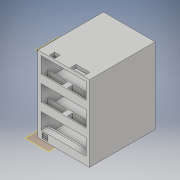
# Autodesk Inventor part: Relé - columnes tapa
Saved by Autodesk Inventor 2019 (Build 230136000, 136)
## iProperties
Created: 2018-08-23
Part Number: Relé - columnes tapa
Material: Genérico
Document SubType Name: Modeling
Designer: Albert Garangou Culebras
Density: 1 g/cm^3
Appearance: Valor por defecto
Author: Albert Garangou Culebras
Autodesk Inventor part; units mm, degrees
ref_plane "YZ Plane" through (0, 0, 0) normal (1, 0, 0) x (0, 1, 0)
ref_plane "XZ Plane" through (0, 0, 0) normal (0, 1, 0) x (-1, 0, 0)
ref_plane "XY Plane" through (0, 0, 0) normal (0, 0, 1) x (1, 0, 0)
ref_plane "Plano de trabajo1" through (0, 3, 0) normal (0, 1, 0) x (1, 0, 0)
ref_plane "Plano de trabajo2" through (4.2498, 73, -5.25) normal (0, 1, 0) x (1, 0, 0)
sketch "Boceto3" plane through (4.2498, 73, -5.25) normal (0, 1, 0) x (1, 0, 0)
  line L0 (37.7502, 51.75) -> (40.7502, 51.75)
  line L1 (-7.2498, -8.25) -> (40.7502, -8.25)
  line L2 (40.7502, -8.25) -> (40.7502, 51.75)
  line L3 (40.7502, 51.75) -> (-7.2498, 51.75)
  line L4 (-7.2498, 51.75) -> (-7.2498, -8.25)
  circle A0 centre (33.5, 43.5) radius 1.25
  circle A1 centre (33.5, 0) radius 1.25
  circle A2 centre (0, 43.5) radius 1.25
  circle A3 centre (0, 0) radius 1.25
  point P0 (-4.2498, -5.25)
  point P1 (37.7502, -5.25)
  point P2 (37.7502, 48.75)
  dimension "d39" = 2.5
  dimension "d40" = 2.5
  dimension "d41" = 2.5
  dimension "d42" = 2.5
  constraints: 10 end point, 4 centre point, 3 coincident, 2 parallel, 1 horizontal, 1 perpendicular
  measures "d39" diameter of A0
  measures "d40" diameter of A1
  measures "d41" diameter of A2
  measures "d42" diameter of A3
ref_plane "Plano de trabajo3" through (4.2498, 73, -5.25) normal (0, -1, 0) x (1, 0, 0)
sketch "Boceto5" plane through (4.2498, 73, -5.25) normal (0, -1, 0) x (1, 0, 0)
  line L0 (-4.2498, 5.25) -> (-4.2498, -48.75) projected
  line L1 (-4.2498, 5.25) -> (-4.2498, -48.75)
  line L2 (37.7502, -48.75) -> (37.7502, 5.25)
  line L3 (37.7502, 5.25) -> (37.7502, 8.25)
  line L4 (37.7502, -48.75) -> (37.7502, -51.75)
  line L5 (-4.2498, 5.25) -> (-7.2498, 5.25)
  line L6 (-4.2498, -48.75) -> (-7.2498, -48.75)
  line L7 (37.7502, -48.75) -> (40.7502, -48.75)
  line L8 (37.7502, 5.25) -> (40.7502, 5.25)
  line L9 (40.7502, 5.25) -> (40.7502, -48.75)
  line L10 (40.7502, -51.75) -> (40.7502, 8.25) projected
  line L11 (-7.2498, -48.75) -> (-7.2498, 5.25)
  line L12 (-7.2498, 8.25) -> (-7.2498, -51.75) projected
  constraints: 20 end point, 2 collinear, 1 horizontal, 1 parallel
extrude "Extrusión5" add sketch "Boceto5" along normal blind 67.5
extrude "Extrusión6" add sketch "Boceto3" along normal blind 3
sketch "Boceto6" plane through (4.2498, 76, -5.25) normal (0, 1, 0) x (1, 0, 0)
  circle A0 centre (0, 43.5) radius 1.25 projected
  circle A1 centre (0, 43.5) radius 1.25
  circle A2 centre (33.5, 43.5) radius 1.25 projected
  circle A3 centre (33.5, 43.5) radius 1.25
  circle A4 centre (33.5, 0) radius 1.25 projected
  circle A5 centre (33.5, 0) radius 1.25
  circle A6 centre (0, 0) radius 1.25
  point P0 (-4.2498, -5.25)
  constraints: 4 centre point, 3 coincident
extrude "Extrusión7" add sketch "Boceto6" against normal blind 3
sketch "Boceto8" plane through (45, 5.5, 0) normal (1, 0, 0) x (0, 0, -1)
  line L0 (0, 0) -> (54, 0) projected
  line L1 (0, 0) -> (54, 0)
  line L2 (54, 0) -> (54, 1.5)
  line L3 (54, 1.5) -> (0, 1.5)
  line L4 (0, 67.5) -> (0, 0) projected
  line L5 (0, 0) -> (0, 1.5)
  line L6 (54, 1.5) -> (54, 21.5)
  line L7 (54, 21.5) -> (54, 22.5)
  line L8 (54, 22.5) -> (0, 22.5)
  line L9 (0, 22.5) -> (0, 24)
  line L10 (0, 24) -> (54, 24)
  line L11 (54, 22.5) -> (54, 24)
  line L12 (54, 24) -> (54, 45)
  line L13 (54, 67.5) -> (54, 0) projected
  line L14 (54, 45) -> (0, 45)
  line L15 (0, 45) -> (0, 46.5)
  line L16 (0, 46.5) -> (54, 46.5)
  line L17 (54, 45) -> (54, 46.5)
  line L18 (54, 67.5) -> (0, 67.5) projected
  line L19 (54, 46.5) -> (54, 67.5)
  point P0 (0, -5.5)
  dimension "d54" = 1.5
  dimension "d55" = 20
  dimension "d60" = 1
  dimension "d61" = 1.5
  dimension "d62" = 21
  dimension "d63" = 1.5
  constraints: 32 end point, 7 perpendicular, 7 point on line, 1 collinear, 1 vertical
  measures "d54" distance of L0.end L2.end
  measures "d55" distance of L2.end L6.end
  measures "d60" distance of L6.end L7.end
  measures "d61" distance of L8.end L9.end
  measures "d62" distance of L10.end L12.end
  measures "d63" distance of L14.end L15.end
extrude "Extrusión8" add sketch "Boceto8" against normal blind 47.25 contours L4 L3 L2 L0 | L4 L10 L11 L8 | L4 L16 L13 L14
sketch "Boceto9" plane through (-3, 5.5, 0) normal (0, 0, 1) x (1, 0, 0)
  line L0 (3, 67.5) -> (3, 46.5) projected
  line L1 (3, 46.5) -> (3, 52.5)
  line L2 (3, 52.5) -> (45, 52.5)
  line L3 (45, 67.5) -> (45, 46.5) projected
  line L4 (45, 52.5) -> (45, 46.5)
  line L5 (45, 46.5) -> (3, 46.5) projected
  line L6 (45, 46.5) -> (3, 46.5)
  line L7 (45, 45) -> (45, 24) projected
  line L8 (3, 24) -> (45, 24)
  line L9 (45, 24) -> (45, 30)
  line L10 (45, 30) -> (3, 30)
  line L11 (3, 30) -> (3, 24)
  line L12 (45, 22.5) -> (45, 1.5) projected
  line L13 (3, 2) -> (3, 1.5)
  line L14 (45, 1.5) -> (3, 1.5) projected
  line L15 (3, 1.5) -> (45, 1.5)
  line L16 (45, 1.5) -> (45, 7.5)
  line L17 (45, 22.5) -> (45, 1.5) projected
  line L18 (45, 7.5) -> (3, 7.5)
  line L19 (45, 7.5) -> (45, 1.5)
  line L20 (3, 1.5) -> (3, 7.5)
  line L21 (3, 22.5) -> (3, 1.5) projected
  point P0 (3, -5.5)
  point P1 (45, 8)
  point P2 (45, 2)
  dimension "d66" = 6
  dimension "d70" = 6
  constraints: 28 end point, 5 collinear, 4 point on line, 2 parallel, 2 perpendicular, 1 horizontal, 1 vertical
  measures "d66" distance of L0.end L1.end
  measures "d70" distance of L12.end L16.end
extrude "Extrusión10" add sketch "Boceto9" along normal blind 1.5
sketch "Boceto11" plane through (-3, 5.5, 0) normal (0, 0, 1) x (1, 0, 0)
  line L0 (48, 0) -> (0, 0) projected
  line L1 (48, 0) -> (0, 0)
  line L2 (0, 0) -> (0, 67.5)
  line L3 (3, 67.5) -> (3, 52.5) projected
  line L4 (0, 67.5) -> (3, 67.5)
  line L5 (3, 67.5) -> (3, 46.5)
  line L6 (45, 46.5) -> (3, 46.5) projected
  line L7 (3, 46.5) -> (45, 46.5)
  line L8 (45, 67.5) -> (45, 52.5) projected
  line L9 (45, 46.5) -> (45, 67.5)
  line L10 (48, 67.5) -> (45, 67.5) projected
  line L11 (45, 67.5) -> (48, 67.5)
  line L12 (48, 67.5) -> (48, 0)
  line L13 (3, 7.5) -> (3, 1.5) projected
  line L14 (3, 22.5) -> (3, 7.5) projected
  line L15 (3, 7.5) -> (3, 22.5)
  line L16 (3, 22.5) -> (45, 22.5)
  line L17 (45, 22.5) -> (45, 1.5) projected
  line L18 (45, 22.5) -> (45, 1.5)
  line L19 (45, 1.5) -> (3, 1.5)
  line L20 (3, 1.5) -> (3, 7.5)
  line L21 (45, 24) -> (3, 24) projected
  line L22 (3, 24) -> (45, 24)
  line L23 (45, 24) -> (45, 45)
  line L24 (3, 45) -> (3, 30) projected
  line L25 (45, 45) -> (3, 45)
  line L26 (3, 45) -> (3, 24)
  point P0 (3, -5.5)
  dimension "d75" = 21
  constraints: 34 end point, 10 perpendicular, 4 collinear, 2 horizontal, 2 point on line, 1 parallel
  measures "d75" distance of L3.start L5.end
extrude "Extrusión12" add sketch "Boceto11" along normal blind 1.5
sketch "Boceto12" plane through (-3, 73, 3) normal (0, 0, 1) x (1, 0, 0)
  line L0 (45, 0) -> (48, 0) projected
  line L1 (0, 3) -> (48, 3)
  line L2 (48, 3) -> (48, 0)
  line L3 (48, 0) -> (0, 0)
  line L4 (0, 0) -> (0, 3)
  point P0 (3, -73)
  constraints: 8 end point, 2 parallel, 1 horizontal, 1 perpendicular
extrude "Extrusión13" cut sketch "Boceto12" against normal blind 1.5
sketch "Boceto13" plane through (45, 73, -57) normal (0, 0, -1) x (-1, 0, 0)
  line L0 (0, 3) -> (48, 3)
  line L1 (48, 3) -> (48, 0)
  line L2 (48, 0) -> (0, 0)
  line L3 (0, 0) -> (0, 3)
  point P0 (45, -73)
  constraints: 8 end point, 2 parallel, 1 horizontal, 1 perpendicular
extrude "Extrusión14" cut sketch "Boceto13" against normal blind 3
sketch "Boceto14" plane through (-3, 5.5, 1.5) normal (0, 0, 1) x (1, 0, 0)
  line L0 (48, 70.5) -> (0, 70.5) projected
  line L1 (0, 0) -> (48, 0) projected
  line L2 (0, 70.5) -> (48, 70.5)
  line L3 (48, 70.5) -> (48, 0)
  line L4 (48, 0) -> (0, 0)
  line L5 (0, 0) -> (0, 70.5)
  line L6 (3, 45) -> (45, 45) projected
  line L7 (3, 45) -> (45, 45)
  line L8 (45, 45) -> (45, 30)
  line L9 (45, 30) -> (3, 30)
  line L10 (3, 30) -> (3, 45)
  line L11 (3, 22.5) -> (45, 22.5) projected
  line L12 (45, 22.5) -> (45, 1.5) projected
  line L13 (3, 22.5) -> (45, 22.5)
  line L14 (45, 22.5) -> (45, 7.5257)
  line L15 (45, 7.5257) -> (3, 7.5257)
  line L16 (3, 7.5257) -> (3, 22.5)
  line L17 (3, 52.5) -> (3, 67.5) projected
  line L18 (45, 67.5) -> (45, 46.5) projected
  line L19 (3, 67.5) -> (45, 67.5)
  line L20 (45, 67.5) -> (45, 52.5)
  line L21 (45, 52.5) -> (3, 52.5)
  line L22 (3, 52.5) -> (3, 67.5)
  point P0 (3, -5.5)
  dimension "d86" = 15
  constraints: 32 end point, 8 parallel, 4 horizontal, 4 perpendicular, 2 point on line
  measures "d86" distance of L19.end L20.end
extrude "Extrusión15" add sketch "Boceto14" along normal blind 5.5
sketch "Boceto15" plane through (0, 58, 0) normal (0, 1, 0) x (1, 0, 0)
  line L0 (42, 0) -> (42, -7)
  line L1 (0, -7) -> (0, 0)
  line L2 (0, -7) -> (1.5, -7)
  line L3 (0, -7) -> (0, -5.5)
  line L4 (0, 0) -> (0, -7) projected
  line L5 (42, -7) -> (42, -6)
  line L6 (42, 0) -> (42, -7) projected
  line L7 (42, -6) -> (0, -6)
  line L8 (0, -7) -> (0, -6)
  line L9 (0, 0) -> (0, -1)
  line L10 (0, -1) -> (42, -1)
  line L11 (42, 0) -> (42, -1)
  dimension "d89" = 1.5
  dimension "d90" = 1.5
  dimension "d91" = 1
  constraints: 20 end point, 5 point on line, 3 perpendicular, 1 collinear, 1 parallel
  measures "d89" distance of L1.start L2.end
  measures "d90" distance of L1.start L3.end
  measures "d91" distance of L0.end L5.end
extrude "Extrusión16" cut sketch "Boceto15" against normal blind 41.75
sketch "Boceto16" plane through (0, 28, 1) normal (0, 0, 1) x (1, 0, 0)
  line L0 (42, 0) -> (0, 0) projected
  line L1 (0, 0) -> (42, 0)
  line L2 (0, 7.5) -> (42, 7.5) projected
  line L3 (21, 0) -> (18.5, 0)
  line L4 (18.5, 0) -> (18.5, 7.5)
  line L5 (18.5, 7.5) -> (23.5, 7.5)
  line L6 (23.5, 7.5) -> (23.5, 0)
  point P0 (0, -28)
  dimension "d94" = 2.5
  dimension "d95" = 5
  constraints: 10 end point, 4 point on line, 2 perpendicular, 1 horizontal, 1 midpoint
  measures "d94" distance of L3.start L3.end
  measures "d95" distance of L4.end L5.end
extrude "Extrusión17" add sketch "Boceto16" along normal blind 5.75
sketch "Boceto17" plane through (0, 58, 1) normal (0, 0, 1) x (1, 0, 0)
  line L0 (0, 0) -> (42, 0) projected
  line L1 (21, 0) -> (18.5, 0)
  line L2 (18.5, 0) -> (23.5, 0)
  line L3 (23.5, 0) -> (23.5, -7.5)
  line L4 (42, -28.5) -> (0, -28.5) projected
  line L5 (23.5, -7.5) -> (18.5, -7.5)
  line L6 (42, -7.5) -> (0, -7.5) projected
  line L7 (18.5, 0) -> (18.5, -7.5)
  point P0 (0, -58)
  dimension "d98" = 2.5
  dimension "d99" = 5
  dimension "d100" = 7.5
  constraints: 10 end point, 3 point on line, 1 midpoint, 1 perpendicular, 1 vertical
  measures "d98" distance of L1.start L1.end
  measures "d99" distance of L1.end L2.end
  measures "d100" distance of L2.end L3.end
extrude "Extrusión18" add sketch "Boceto17" along normal blind 5.75
sketch "Boceto18" plane through (4.2498, 76, -5.25) normal (0, 1, 0) x (1, 0, 0)
  line L0 (-4.2498, 48.75) -> (-4.2498, -12.25) projected
  line L1 (-4.2498, -12.25) -> (-4.2498, -11.25)
  line L2 (-4.2498, -11.25) -> (-4.2498, -6.25)
  line L3 (2.5002, -11.25) -> (7.5002, -11.25)
  line L4 (-4.2498, -5.25) -> (-4.2498, 48.75) projected
  line L5 (7.5002, -11.25) -> (7.5002, -6.25)
  line L6 (2.5002, -11.25) -> (2.5002, -6.25)
  line L7 (2.5002, -6.25) -> (7.5002, -6.25)
  line L8 (23.5002, -6.25) -> (23.5002, -11.25)
  line L9 (33.5002, -6.25) -> (33.5002, -11.25)
  line L10 (23.5002, -6.25) -> (33.5002, -6.25)
  line L11 (23.5002, -11.25) -> (33.5002, -11.25)
  dimension "d103" = 1
  dimension "d104" = 5
  constraints: 20 end point, 2 horizontal, 2 point on line, 1 perpendicular, 1 vertical
  measures "d103" distance of L0.end L1.end
  measures "d104" distance of L1.end L2.end
extrude "Extrusión19" cut sketch "Boceto18" against normal blind 6
sketch "Boceto19" plane through (4.2498, 76, -5.25) normal (0, 1, 0) x (1, 0, 0)
  line L0 (23.5002, -6.25) -> (33.5002, -6.25) projected
  line L1 (23.5002, -6.25) -> (22.2502, -6.25)
  line L2 (37.7502, -6.25) -> (19.2502, -6.25) projected
  line L3 (23.5002, -11.25) -> (22.2502, -11.25)
  line L4 (19.2502, -11.25) -> (37.7502, -11.25) projected
  line L5 (22.2502, -6.25) -> (22.2502, -11.25)
  line L6 (-4.2498, -6.75) -> (37.7502, -6.75) projected
  line L7 (33.5002, -6.25) -> (35, -6.25)
  line L8 (35, -11.25) -> (35, -6.25)
  line L9 (23.5002, -11.25) -> (33.5002, -11.25) projected
  line L10 (35, -11.25) -> (33.5002, -11.25)
  point P0 (-4.2498, -5.25)
  dimension "d115" = 1.25
  constraints: 12 end point, 4 point on line, 2 perpendicular, 1 horizontal
  measures "d115" distance of L0.start L1.end
extrude "Extrusión20" cut sketch "Boceto19" against normal blind 9.5
sketch "Boceto20" plane through (-3, 5.5, 7) normal (0, 0, 1) x (1, 0, 0)
  line L0 (3, 7.5) -> (3, 7.5257) projected
  line L1 (45, 1.5) -> (3, 1.5) projected
  line L2 (4.2634, 4.6029) -> (9.2628, 4.6029)
  line L3 (4.2634, 2.9329) -> (9.2628, 2.9329)
  line L4 (4.2634, 3.1329) -> (9.2628, 3.1329)
  line L5 (4.2634, 4.8029) -> (9.2628, 4.8029)
  line L6 (4.2634, 4.8029) -> (4.2634, 6.2729)
  line L7 (4.2634, 6.2729) -> (9.2628, 6.2729)
  line L8 (9.2628, 2.9329) -> (9.2628, 1.4629)
  line L9 (9.2628, 1.4629) -> (4.2634, 1.4629)
  line L10 (4.2634, 1.4629) -> (4.2634, 2.9329)
  line L11 (4.2634, 3.1329) -> (4.2634, 4.6029)
  line L12 (9.2628, 4.8029) -> (9.2628, 6.2729)
  line L13 (9.2628, 4.6029) -> (9.2628, 3.1329)
  point P0 (3, -5.5)
  dimension "d135" = 1.47
  constraints: 24 end point, 3 vertical, 1 perpendicular
  measures "d135" distance of L3.end L8.end
extrude "Extrusión21" cut sketch "Boceto20" against normal blind 1
sketch "Boceto21" plane through (-3, 5.5, 7) normal (0, 0, 1) x (1, 0, 0)
  line L0 (4.2634, 6.2729) -> (9.2628, 6.2729) projected
  line L1 (4.2634, 6.2729) -> (9.2628, 6.2729)
  line L2 (9.2628, 2.9329) -> (9.2628, 1.4629) projected
  line L3 (9.2628, 6.2729) -> (9.2628, 1.4629)
  line L4 (9.2628, 1.4629) -> (4.2634, 1.4629) projected
  line L5 (9.2628, 1.4629) -> (4.2634, 1.4629)
  line L6 (4.2634, 4.8029) -> (4.2634, 6.2729) projected
  line L7 (4.2634, 1.4629) -> (4.2634, 6.2729)
  line L8 (4.2634, 6.2729) -> (4.0634, 6.2729)
  line L9 (4.0634, 6.2729) -> (4.0634, 1.4629)
  line L10 (45, 1.5) -> (3, 1.5) projected
  line L11 (4.0634, 1.4629) -> (4.2634, 1.4629)
  line L12 (9.2628, 6.2729) -> (9.2628, 4.8029) projected
  line L13 (9.2628, 6.2729) -> (9.4628, 6.2729)
  line L14 (9.4628, 6.2729) -> (9.4628, 1.4629)
  line L15 (9.4628, 1.4629) -> (9.2628, 1.4629)
  point P0 (3, -5.5)
  dimension "d138" = 0.2
  dimension "d139" = 0.2
  constraints: 20 end point, 6 perpendicular, 3 collinear, 1 horizontal
  measures "d138" distance of L0.start L8.end
  measures "d139" distance of L0.end L13.end
extrude "Extrusión22" cut sketch "Boceto21" against normal blind 1 contours L6 L7 L10 L9 L8 | L13 L14 L10 L2 L3 | L7 L11 L9 L10 | L14 L15 L2 L10
sketch "Boceto22" plane through (-3, 5.5, 7) normal (0, 0, 1) x (1, 0, 0)
  line L0 (4.2634, 4.8029) -> (4.2634, 4.6029) projected
  line L1 (4.2634, 4.7029) -> (4.7634, 4.7029) construction
  line L2 (4.2634, 4.7029) -> (4.2634, 4.9529)
  line L3 (4.2634, 4.7029) -> (4.2634, 4.4529)
  line L4 (4.2634, 4.4529) -> (9.2628, 4.4529)
  line L5 (4.2634, 4.6029) -> (9.2628, 4.6029) projected
  line L6 (9.2628, 4.4529) -> (9.2628, 4.9529)
  line L7 (9.2628, 4.6029) -> (9.2628, 4.8029) projected
  line L8 (9.2628, 4.9529) -> (4.2634, 4.9529)
  line L9 (4.2634, 3.1329) -> (4.2634, 2.9329) projected
  line L10 (4.2634, 3.0329) -> (4.2634, 3.2829)
  line L11 (4.2634, 3.2829) -> (9.2628, 3.2829)
  line L12 (9.2628, 3.2829) -> (9.2628, 2.7829)
  line L13 (9.2628, 2.7829) -> (4.2634, 2.7829)
  line L14 (4.2634, 2.7829) -> (4.2634, 3.0329)
  point P0 (3, -5.5)
  dimension "d148" = 0.5
  dimension "d149" = 0.25
  dimension "d150" = 0.5
  constraints: 22 end point, 4 perpendicular, 2 collinear, 2 midpoint, 2 vertical, 1 horizontal, 1 parallel, 1 point on line
  measures "d148" distance of L4.end L6.end
  measures "d149" distance of L10.start L10.end
  measures "d150" distance of L11.end L12.end
extrude "Extrusión23" add sketch "Boceto22" against normal blind 1
